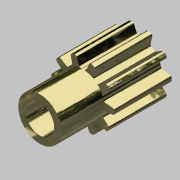
# Autodesk Inventor part: small_gear
Saved by Autodesk Inventor 2019.3 (Build 233278000, 278)
## iProperties
Created: 2019-04-17
Part Number: small_gear
Material: Generic
Document SubType Name: Modeling
Designer: Varga Daniel
Density: 1 g/cm^3
Appearance: Gold - Metal
Author: Varga Daniel
Autodesk Inventor part; units mm, degrees
ref_plane "YZ Plane" through (0, 0, 0) normal (1, 0, 0) x (0, 1, 0)
ref_plane "XZ Plane" through (0, 0, 0) normal (0, 1, 0) x (-1, 0, 0)
ref_plane "XY Plane" through (0, 0, 0) normal (0, 0, 1) x (1, 0, 0)
sketch "Sketch1" plane through (0, 0, 0) normal (0, 0, 1) x (1, 0, 0)
  circle A0 centre (0, 0) radius 1.5
  dimension "d0" = 3
  constraints: 1 centre point, 1 coincident
  measures "d0" diameter of A0
extrude "Extrusion1" add sketch "Sketch1" along normal blind 7
sketch "Sketch2" plane through (0, 0, 0) normal (0, 0, -1) x (-1, 0, 0)
  line L0 (0, 0) -> (2.853, 0) construction
  line L1 (0, 0) -> (0, -3.3556) construction
  line L2 (2.2, 0) -> (2.2, -0.063)
  line L3 (2.0636, -0.2124) -> (0, -0.4)
  circle A0 centre (0, 0) radius 1.5 projected
  line L4 (0, -0.4) -> (0, 0)
  line L5 (2.2, 0) -> (0, 0)
  line L6 (2.2, 0) -> (2.2, 0.063)
  line L7 (2.0636, 0.2124) -> (0, 0.4)
  line L8 (0, 0.4) -> (0, 0)
  arc A1 (2.2, 0.063) -> (2.0636, 0.2124) centre (2.05, 0.063) ccw
  arc A2 (2.0636, -0.2124) -> (2.2, -0.063) centre (2.05, -0.063) ccw
  line L9 (1.7798, 1.2931) -> (1.8169, 1.2421)
  line L10 (1.7943, 1.0411) -> (0.2351, -0.3236)
  line L11 (0.2351, -0.3236) -> (0, 0)
  line L12 (1.7798, 1.2931) -> (0, 0)
  line L13 (1.7798, 1.2931) -> (1.7428, 1.3441)
  line L14 (1.5446, 1.3848) -> (-0.2351, 0.3236)
  line L15 (-0.2351, 0.3236) -> (0, 0)
  arc A3 (1.7428, 1.3441) -> (1.5446, 1.3848) centre (1.6214, 1.2559) ccw
  arc A4 (1.7943, 1.0411) -> (1.8169, 1.2421) centre (1.6955, 1.154) ccw
  line L16 (0.6798, 2.0923) -> (0.7398, 2.0729)
  line L17 (0.8397, 1.8969) -> (0.3804, -0.1236)
  line L18 (0.3804, -0.1236) -> (0, 0)
  line L19 (0.6798, 2.0923) -> (0, 0)
  line L20 (0.6798, 2.0923) -> (0.6199, 2.1118)
  line L21 (0.4357, 2.0282) -> (-0.3804, 0.1236)
  line L22 (-0.3804, 0.1236) -> (0, 0)
  arc A5 (0.6199, 2.1118) -> (0.4357, 2.0282) centre (0.5736, 1.9691) ccw
  arc A6 (0.8397, 1.8969) -> (0.7398, 2.0729) centre (0.6934, 1.9302) ccw
  line L23 (-0.6798, 2.0923) -> (-0.6199, 2.1118)
  line L24 (-0.4357, 2.0282) -> (0.3804, 0.1236)
  line L25 (0.3804, 0.1236) -> (0, 0)
  line L26 (-0.6798, 2.0923) -> (0, 0)
  line L27 (-0.6798, 2.0923) -> (-0.7398, 2.0729)
  line L28 (-0.8397, 1.8969) -> (-0.3804, -0.1236)
  line L29 (-0.3804, -0.1236) -> (0, 0)
  arc A7 (-0.7398, 2.0729) -> (-0.8397, 1.8969) centre (-0.6934, 1.9302) ccw
  arc A8 (-0.4357, 2.0282) -> (-0.6199, 2.1118) centre (-0.5736, 1.9691) ccw
  line L30 (-1.7798, 1.2931) -> (-1.7428, 1.3441)
  line L31 (-1.5446, 1.3848) -> (0.2351, 0.3236)
  line L32 (0.2351, 0.3236) -> (0, 0)
  line L33 (-1.7798, 1.2931) -> (0, 0)
  line L34 (-1.7798, 1.2931) -> (-1.8169, 1.2421)
  line L35 (-1.7943, 1.0411) -> (-0.2351, -0.3236)
  line L36 (-0.2351, -0.3236) -> (0, 0)
  arc A9 (-1.8169, 1.2421) -> (-1.7943, 1.0411) centre (-1.6955, 1.154) ccw
  arc A10 (-1.5446, 1.3848) -> (-1.7428, 1.3441) centre (-1.6214, 1.2559) ccw
  line L37 (-2.2, 0) -> (-2.2, 0.063)
  line L38 (-2.0636, 0.2124) -> (0, 0.4)
  line L39 (0, 0.4) -> (0, 0)
  line L40 (-2.2, 0) -> (0, 0)
  line L41 (-2.2, 0) -> (-2.2, -0.063)
  line L42 (-2.0636, -0.2124) -> (0, -0.4)
  line L43 (0, -0.4) -> (0, 0)
  arc A11 (-2.2, -0.063) -> (-2.0636, -0.2124) centre (-2.05, -0.063) ccw
  arc A12 (-2.0636, 0.2124) -> (-2.2, 0.063) centre (-2.05, 0.063) ccw
  line L44 (-1.7798, -1.2931) -> (-1.8169, -1.2421)
  line L45 (-1.7943, -1.0411) -> (-0.2351, 0.3236)
  line L46 (-0.2351, 0.3236) -> (0, 0)
  line L47 (-1.7798, -1.2931) -> (0, 0)
  line L48 (-1.7798, -1.2931) -> (-1.7428, -1.3441)
  line L49 (-1.5446, -1.3848) -> (0.2351, -0.3236)
  line L50 (0.2351, -0.3236) -> (0, 0)
  arc A13 (-1.7428, -1.3441) -> (-1.5446, -1.3848) centre (-1.6214, -1.2559) ccw
  arc A14 (-1.7943, -1.0411) -> (-1.8169, -1.2421) centre (-1.6955, -1.154) ccw
  line L51 (-0.6798, -2.0923) -> (-0.7398, -2.0729)
  line L52 (-0.8397, -1.8969) -> (-0.3804, 0.1236)
  line L53 (-0.3804, 0.1236) -> (0, 0)
  line L54 (-0.6798, -2.0923) -> (0, 0)
  line L55 (-0.6798, -2.0923) -> (-0.6199, -2.1118)
  line L56 (-0.4357, -2.0282) -> (0.3804, -0.1236)
  line L57 (0.3804, -0.1236) -> (0, 0)
  arc A15 (-0.6199, -2.1118) -> (-0.4357, -2.0282) centre (-0.5736, -1.9691) ccw
  arc A16 (-0.8397, -1.8969) -> (-0.7398, -2.0729) centre (-0.6934, -1.9302) ccw
  line L58 (0.6798, -2.0923) -> (0.6199, -2.1118)
  line L59 (0.4357, -2.0282) -> (-0.3804, -0.1236)
  line L60 (-0.3804, -0.1236) -> (0, 0)
  line L61 (0.6798, -2.0923) -> (0, 0)
  line L62 (0.6798, -2.0923) -> (0.7398, -2.0729)
  line L63 (0.8397, -1.8969) -> (0.3804, 0.1236)
  line L64 (0.3804, 0.1236) -> (0, 0)
  arc A17 (0.7398, -2.0729) -> (0.8397, -1.8969) centre (0.6934, -1.9302) ccw
  arc A18 (0.4357, -2.0282) -> (0.6199, -2.1118) centre (0.5736, -1.9691) ccw
  line L65 (1.7798, -1.2931) -> (1.7428, -1.3441)
  line L66 (1.5446, -1.3848) -> (-0.2351, -0.3236)
  line L67 (-0.2351, -0.3236) -> (0, 0)
  line L68 (1.7798, -1.2931) -> (0, 0)
  line L69 (1.7798, -1.2931) -> (1.8169, -1.2421)
  line L70 (1.7943, -1.0411) -> (0.2351, 0.3236)
  line L71 (0.2351, 0.3236) -> (0, 0)
  arc A19 (1.8169, -1.2421) -> (1.7943, -1.0411) centre (1.6955, -1.154) ccw
  arc A20 (1.5446, -1.3848) -> (1.7428, -1.3441) centre (1.6214, -1.2559) ccw
  point P0 (2.2, -0.2)
  point P1 (2.2, 0.2)
  point P2 (1.8974, 1.1313)
  point P3 (1.6623, 1.4549)
  point P4 (0.87, 2.0305)
  point P5 (0.4896, 2.1541)
  point P6 (-0.4896, 2.1541)
  point P7 (-0.87, 2.0305)
  point P8 (-1.6623, 1.4549)
  point P9 (-1.8974, 1.1313)
  point P10 (-2.2, 0.2)
  point P11 (-2.2, -0.2)
  point P12 (-1.8974, -1.1313)
  point P13 (-1.6623, -1.4549)
  point P14 (-0.87, -2.0305)
  point P15 (-0.4896, -2.1541)
  point P16 (0.4896, -2.1541)
  point P17 (0.87, -2.0305)
  point P18 (1.6623, -1.4549)
  point P19 (1.8974, -1.1313)
  dimension "d3" = 0.2
  dimension "d5" = 0.7
  dimension "d6" = 0.4
  dimension "d7" = 0.15
  dimension "d10" = 360
  constraints: 144 end point, 42 point on line, 40 point on circle, 20 centre point, 4 tangent, 2 coincident, 2 collinear, 2 symmetric about line, 2 vertical, 1 equal radius, 1 horizontal, 219 other
  measures "d3" distance of L2.start point (2.2, -0.2)
  measures "d5" distance edge to line of A0 L2
  measures "d6" distance of L3.end L0.start
  measures "d7" radius of A1
extrude "Extrusion2" add sketch "Sketch2" against normal blind 4 contours L2 A2 L3 A0 L5 | L5 A0 L7 A1 L6 | L5 L10 L7 A0 | A0 L3 L70 L5 | L10 L63 L5 | L70 L17 L7 L10 | L70 L3 L63 L10 | L5 L17 L70 | L10 L7 L12 A0 | A0 L12 L9 A4 L10 | L70 A0 L68 L3 | L70 A19 L69 L68 A0 | L17 L18 L5 | L63 L24 L70 L17 | L63 L10 L56 L17 | L5 L25 L63 | L63 L68 L10 | L70 L12 L17 | L12 L17 L14 A0 | A0 L14 A3 L13 L12 | L12 L24 L7 | L7 L24 L14 L17 | L63 L66 L56 L3 | L68 A0 L66 L63 | L3 L56 L68 | L68 L65 A20 L66 A0 | L61 L3 L4 | L26 L38 L8 | L68 L10 L11 | L32 L70 L12 | L33 L45 L15 | L8 L7 L19 | L40 L52 L22 | L12 L24 L25 | L15 L14 L26 | L47 L59 L29 | L19 L31 L32 | L22 L21 L33 | L54 L66 L36 | L29 L28 L40 | L36 L35 L47 | L4 L42 L54 | L11 L49 L61 | L18 L56 L68 | L56 L3 L49 L10 | L70 L31 L7 L24 | L7 L19 L24 | L14 L19 A0 L17 | L56 L61 L3 | L63 A0 L61 L66 | L3 L49 L66 L42 | L38 L14 L31 L7 | L45 L21 L38 L14 | L31 L14 L19 | L52 L28 L45 L21 | L26 L31 L14 | L38 L21 L26 | L59 L35 L52 L28 | L33 L38 L21 | L45 L28 L33 | L66 L42 L59 L35 | L40 L45 L28 | L52 L35 L40 | L47 L52 L35 | L59 L42 L47 | L54 L59 L42 | L66 L49 L54 | L61 L66 L49 | A0 L19 L16 A6 L17 | L24 L21 A0 L19 | L14 L31 L21 L24 | L61 A0 L59 L56 | L56 L59 L49 L66 | L63 A17 L62 L61 A0 | L26 A0 L24 L21 | L31 L28 A0 L26 | L21 L38 L28 L31 | L33 A0 L31 L28 | L38 L35 A0 L33 | L28 L45 L35 L38 | L40 A0 L38 L35 | L45 L42 A0 L40 | L35 L52 L42 L45 | L47 A0 L45 L42 | L52 L49 A0 L47 | L42 L59 L49 L52 | L54 A0 L52 L49 | L59 L56 A0 L54 | A0 L21 A5 L20 L19 | L61 L58 A18 L59 A0 | L26 L23 A8 L24 A0 | A0 L28 A7 L27 L26 | L33 L30 A10 L31 A0 | A0 L35 A9 L34 L33 | L40 L37 A12 L38 A0 | A0 L42 A11 L41 L40 | L47 L44 A14 L45 A0 | A0 L49 A13 L48 L47 | L54 L51 A16 L52 A0 | A0 L56 A15 L55 L54
fillet "Fillet1" radius 0.15 20 edges at (-0.709, -1.3219, 2) (-1.0381, -1.0828, 2) (-1.3506, -0.6527, 2) (-1.4763, 0.2658, 2) (-1.4763, -0.2658, 2) (0.2034, -1.4861, 2) (-0.709, 1.3219, 2) (-1.3506, 0.6527, 2) (-0.2034, 1.4861, 2) (0.709, 1.3219, 2) (1.4763, 0.2658, 2) (1.0381, -1.0828, 2) (1.4763, -0.2658, 2) (1.3506, 0.6527, 2) (1.0381, 1.0828, 2) (0.2034, 1.4861, 2) (-1.0381, 1.0828, 2) (1.3506, -0.6527, 2) (0.709, -1.3219, 2) (-0.2034, -1.4861, 2)
sketch "Sketch3" plane through (0, 0, 7) normal (0, 0, 1) x (1, 0, 0)
  circle A0 centre (0, 0) radius 1.5 projected
  circle A1 centre (0, 0) radius 1
  dimension "d15" = 2
  constraints: 1 centre point, 1 coincident
  measures "d15" diameter of A1
extrude "Extrusion3" cut sketch "Sketch3" against normal through all contours A1
body "Solid1"
